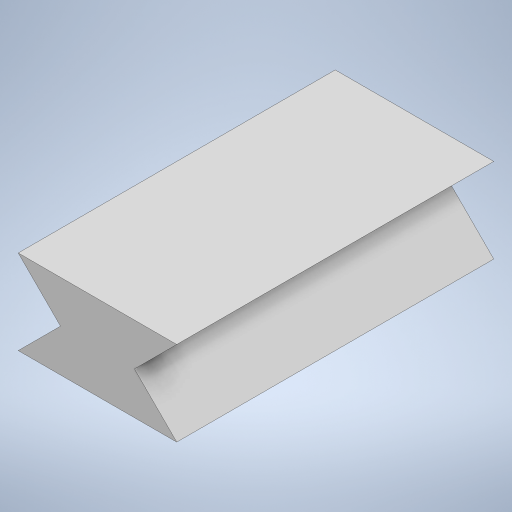
# Autodesk Inventor part: Verbindungsstück_RescueErhöhungen
Saved by Autodesk Inventor 2024 (Build 280153000, 153)
## iProperties
Created: 2025-02-21
Part Number: Verbindungsstück_RescueErhöhungen
Material: Generisch
Document SubType Name: Sheet Metal
Designer: Carla
Density: 1 g/cm^3
Sheet Metal Rule: Standard_mm
Appearance: Vorgabe
Author: Carla
Autodesk Inventor part; units mm, degrees
ref_plane "YZ Plane" through (0, 0, 0) normal (1, 0, 0) x (0, 1, 0)
ref_plane "XZ Plane" through (0, 0, 0) normal (0, 1, 0) x (-1, 0, 0)
ref_plane "XY Plane" through (0, 0, 0) normal (0, 0, 1) x (1, 0, 0)
sketch "Skizze1" plane through (0, 0, 0) normal (0, 1, 0) x (-1, 0, 0)
  line L0 (7.5, 4) -> (-7.5, 4)
  line L1 (3.5, 0) -> (-3.5, 0)
  line L2 (7.5, 4) -> (3.5, 0)
  line L3 (-7.5, 4) -> (-3.5, 0)
  line L4 (11.5, 0) -> (-11.041, 0) construction
  line L5 (-7.5, -4) -> (-3.5, 0)
  line L6 (-7.5, -4) -> (7.5, -4)
  line L7 (7.5, -4) -> (3.5, 0)
  point P0 (0, 0)
  point P1 (0, 0)
  point P2 (-3.5, 0)
  dimension "d1" = 15
  dimension "d3" = 7
  dimension "d4" = 3.5
  dimension "d5" = 7.5
  dimension "d8" = 360
  constraints: 16 end point, 4 horizontal, 1 midpoint, 15 other
  measures "d1" distance of L0.start L0.end
  measures "d3" distance of L1.start L1.end
  measures "d4" distance of point (0, 0) L1.start
  measures "d5" horizontal distance of point (0, 0) L0.start
extrude "Extrusion1" add sketch "Skizze1" along normal blind 30
equation "\"Biegeradius\" = Stärke"
equation "\"BreiteBiegungsfreistellung\" = Stärke"
equation "\"TiefeBiegungsfreistellung\" = 0.5 * Stärke"
equation "\"GrößeEckenfreistellung\" = 4 * Stärke"
equation "\"MinimalRest\" = 2 * Stärke"
equation "\"Übergangsradius\" = Biegeradius"
equation "\"JacobiRadiusGröße\" = Biegeradius"
equation "\"Abstandsgröße\" = Stärke"
equation "\"Stärke\" = 0.5"
